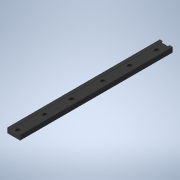
# Autodesk Inventor part: Rail
Saved by Autodesk Inventor 2021 (Build 250183000, 183)
## iProperties
Created: 2024-02-17
Part Number: Rail
Material: Generic
Document SubType Name: Modeling
Designer: Lukas
Density: 1 g/cm^3
Appearance: Default
Author: Lukas
Autodesk Inventor part; units mm, degrees
ref_plane "YZ Plane" through (0, 0, 0) normal (1, 0, 0) x (0, 1, 0)
ref_plane "XZ Plane" through (0, 0, 0) normal (0, 1, 0) x (-1, 0, 0)
ref_plane "XY Plane" through (0, 0, 0) normal (0, 0, 1) x (1, 0, 0)
sketch "Sketch1" plane through (0, 0, 0) normal (0, 0, 1) x (1, 0, 0)
  line L0 (-4, 2.75) -> (-7, 2.75)
  line L1 (-7, 2.75) -> (-7, -2.75)
  line L2 (-7, -2.75) -> (7, -2.75)
  line L3 (7, -2.75) -> (7, 2.75)
  line L4 (7, 2.75) -> (4, 2.75)
  line L5 (4, 2.75) -> (5, 0.75)
  line L6 (5, 0.75) -> (-5, 0.75)
  line L7 (-5, 0.75) -> (-4, 2.75)
  point P0 (0, 0)
  point P1 (0, 0.75)
  point P2 (0, -2.75)
  point P3 (-7, 0)
  dimension "d0" = 14
  dimension "d2" = 3.5
  dimension "d4" = 10
  dimension "d19" = 5.5
  dimension "d20" = 8
  constraints: 16 end point, 3 midpoint, 3 perpendicular, 2 equal length, 2 point on line, 2 vertical alignment, 1 horizontal, 1 horizontal alignment, 1 parallel
  measures "d0" distance between parallel lines of L3 L1
  measures "d2" distance between parallel lines of L2 L6
  measures "d4" distance of L5.end L6.end
  measures "d19" distance of L0.end L1.end
  measures "d20" distance of L4.end L0.start
extrude "Extrusion1" add sketch "Sketch1" against normal mid plane 170
sketch "Sketch2" plane through (-7, -2.75, -85) normal (0, -1, 0) x (1, 0, 0)
  circle A0 centre (7, 165) radius 1.6
  circle A1 centre (7, 135) radius 1.6
  circle A2 centre (7, 105) radius 1.6
  circle A3 centre (7, 70) radius 1.6
  circle A4 centre (7, 40) radius 1.6
  circle A5 centre (7, 10) radius 1.6
  point P0 (7, 85)
  dimension "d7" = 3.2
  dimension "d8" = 15
  dimension "d9" = 20
  dimension "d10" = 30
  dimension "d11" = 30
  dimension "d12" = 30
  dimension "d13" = 30
  constraints: 6 centre point, 6 vertical alignment, 5 equal radius
  measures "d7" diameter of A5
  measures "d8" distance of A3.centre point (7, 85)
  measures "d9" distance of A2.centre point (7, 85)
  measures "d10" distance of A4.centre A3.centre
  measures "d11" distance of A5.centre A4.centre
  measures "d12" distance of A2.centre A1.centre
  measures "d13" distance of A1.centre A0.centre
extrude "Extrusion2" cut sketch "Sketch2" against normal through all
sketch "Sketch3" plane through (-5, 0.75, -85) normal (0, 1, 0) x (1, 0, 0)
  circle A0 centre (5, -165) radius 1.6 projected
  circle A1 centre (5, -135) radius 1.6 projected
  circle A2 centre (5, -135) radius 1.6 projected
  circle A3 centre (5, -105) radius 1.6 projected
  circle A4 centre (5, -105) radius 1.6 projected
  circle A5 centre (5, -70) radius 1.6 projected
  circle A6 centre (5, -40) radius 1.6 projected
  circle A7 centre (5, -10) radius 1.6 projected
  circle A8 centre (5, -165) radius 3
  circle A9 centre (5, -135) radius 3
  circle A10 centre (5, -105) radius 1.6 projected
  circle A11 centre (5, -105) radius 3
  circle A12 centre (5, -70) radius 1.6 projected
  circle A13 centre (5, -70) radius 3
  circle A14 centre (5, -40) radius 3
  circle A15 centre (5, -10) radius 1.6 projected
  circle A16 centre (5, -10) radius 3
  point P0 (5, -85)
  dimension "d16" = 6
  constraints: 6 centre point, 6 coincident, 5 equal radius
  measures "d16" diameter of A8
extrude "Extrusion3" cut sketch "Sketch3" against normal blind 2.5 contours A0 | A1 | A3 | A5 | A6 | A7 | A8 | A9 | A11 | A13 | A14 | A16
equation "\"d11\" = d10"
equation "\"d12\" = d10"
equation "\"d13\" = d10"
body "Solid1"
